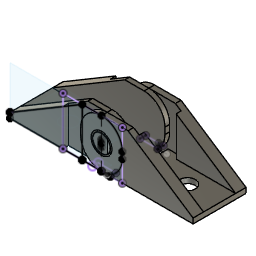
chain-link-ends (Autodesk Fusion 360 design; units mm, degrees)
Autodesk Fusion 360 part; units mm, degrees
note: some values were not read from the file. Set by a fixed rule: which sketch regions a step uses.
sketch "Sketch1" plane through (0, 0, 0) normal (0, 0, 1) x (1, 0, 0)
  line L0 (0, 0) -> (35, 0)
  line L1 (35, 0) -> (35, 16.5)
  line L2 (35, 16.5) -> (0, 16.5)
  line L3 (0, 16.5) -> (0, 0)
  line L4 (0, 14.75) -> (16.5, 14.75)
  line L5 (16.5, 14.75) -> (16.5, 13.25)
  line L6 (16.5, 13.25) -> (35, 13.25)
  line L7 (0, 1.75) -> (16.5, 1.75)
  line L8 (16.5, 1.75) -> (16.5, 3.25)
  line L9 (16.5, 3.25) -> (35, 3.25)
  line L10 (6.5, 16.5) -> (6.5, 0) construction
  line L11 (0, 8.25) -> (35, 8.25) construction
  line L12 (16.5, 14.75) -> (16.5, 16.5) construction
  line L13 (16.5, 1.75) -> (16.5, 0) construction
  line L14 (12.5, 14.75) -> (12.5, 1.75)
  circle A0 centre (25, 8.25) radius 2.5
  dimension "d1" = 35
  dimension "d2" = 16.5
  dimension "d3" = 6.5
  dimension "d4" = 10
  dimension "d5" = 10
  dimension "d7" = 13
  dimension "d9" = 10
  dimension "d10" = 6
  dimension "d11" = 5
  dimension "d12" = 10
  constraint horizontal L0
  constraint vertical L1
  constraint horizontal L2
  constraint vertical L3
  constraint coincident L0.start L3.end
  constraint coincident L3 L4.start
  constraint perpendicular L3 L4
  constraint perpendicular L4 L5
  constraint coincident L1 L6.end
  constraint perpendicular L1 L6
  constraint coincident L3 L7.start
  constraint perpendicular L3 L7
  constraint perpendicular L6 L8
  constraint coincident L1 L9.end
  constraint perpendicular L1 L9
  constraint coincident L2 L10.start
  constraint coincident L0 L10.end
  constraint perpendicular L0 L10
  constraint midpoint L3 L11.start
  constraint midpoint L1 L11.end
  constraint coincident L2 L12.end
  constraint perpendicular L2 L12
  constraint coincident L0 L13.end
  constraint perpendicular L0 L13
  constraint equal L12 L13
  constraint equal L5 L8
  constraint coincident L4 L14.start
  constraint coincident L7 L14.end
  constraint perpendicular L7 L14
  constraint coincident L11 A0.centre
  measures "d1" distance of L0.start L0.end
  measures "d2" distance of L0.start L2.end
  measures "d3" distance of L3 L10
  measures "d4" distance of L5 L10
  measures "d5" distance of L8 L10
  measures "d7" distance of L4 L7
  measures "d9" distance of L6 L9
  measures "d10" distance of L10 L14
  measures "d11" diameter of A0
  measures "d12" distance of L1 A0.centre
extrude "Extrude1" add sketch "Sketch1" along normal blind 1.6 contours L1 L4 L5 L6 L7 L8 L9 L14 makes body 1
extrude "Extrude2" add sketch "Sketch1" along normal blind 15 contours L0 L1 L3 L7 L8 L9 | L1 L2 L3 L4 L5 L6 bodies 1
sketch "Sketch2" plane through (0, 0, 0) normal (0, -1, 0) x (1, 0, 0)
  line L0 (0, 0) -> (35, 0)
  line L1 (35, 0) -> (35, 15)
  line L2 (35, 15) -> (0, 15)
  line L3 (0, 15) -> (0, 0)
  line L4 (0, 8.5) -> (0, 6.5)
  arc A0 (0, 6.5) -> (6.5, 0) centre (6.5, 6.5) ccw
  arc A1 (6.5, 15) -> (0, 8.5) centre (6.5, 8.5) ccw
  line L5 (6.5, 15) -> (14.7505, 15)
  line L6 (14.7505, 15) -> (35, 1.6)
  line L7 (35, 1.6) -> (35, 0)
  line L8 (6.5, 0) -> (35, 0)
  line L9 (0, 0) -> (35, 0)
  circle A2 centre (6.5, 7.5) radius 3.25
  line L10 (22.5, 1.6) -> (27.5, 1.6)
  line L11 (16.5, 1.6) -> (12.5, 1.6)
  line L12 (12.5, 1.6) -> (16.5, 1.6)
  line L13 (16.5, 1.6) -> (35, 1.6)
  line L14 (35, 1.6) -> (16.5, 1.6)
  line L15 (6.5, 0) -> (6.5, 15)
  point P0 (6.5, 0)
  dimension "d17" = 6.5
  constraint coincident L3 L4.start
  constraint coincident L3 L4.end
  constraint coincident L0 P0
  constraint tangent L4 A0
  constraint coincident L2 A1.start
  constraint tangent L4 A1
  constraint coincident L2 L5.end
  constraint parallel L2 L5
  constraint coincident L1 L6.end
  constraint coincident L0.end L1.start
  constraint tangent A0 L9
  constraint tangent A1 L5
  constraint coincident P0 A0.end
  constraint coincident L5 A1.start
  constraint vertical L15
  constraint coincident A2.centre L15
  constraint midpoint A2.centre L15
  constraint equal A0 A1
  constraint coincident L6.end L7.start
  measures "d17" diameter of A2
extrude "Extrude3" cut sketch "Sketch2" against normal up to surface (16.5 mm away) contours L0 L3 A0 L9 | A2 L15 | A2 L15 | L2 L3 A1 | L1 L2 L6 bodies 1
copy_body "Body->Comp1" bodies 1 removing the originals makes body 2 in component "end-1"
sketch "Sketch1 (2)" plane through (0, 0, 0) normal (0, 0, 1) x (1, 0, 0) in component "end-2"
  circle A0 centre (10, 8.25) radius 2.5
  line L0 (0, 8.25) -> (35, 8.25) construction
  line L1 (0, 16.5) -> (0, 0)
  line L2 (16.5, 13.25) -> (35, 13.25)
  line L3 (16.5, 14.75) -> (16.5, 16.5) construction
  line L4 (28.5, 14.75) -> (28.5, 1.75) construction
  line L5 (16.5, 1.75) -> (16.5, 0) construction
  line L6 (16.5, 3.25) -> (35, 3.25)
  line L7 (35, 14.75) -> (16.5, 14.75)
  line L8 (16.5, 14.75) -> (16.5, 15.0527)
  line L9 (16.5, 16.5) -> (16.5, 14.75)
  line L10 (16.5, 16.5) -> (0, 16.5)
  line L11 (16.5, 13.25) -> (0, 13.25)
  line L12 (16.5, 3.25) -> (0, 3.25)
  line L13 (16.5, 1.75) -> (35, 1.75)
  line L14 (16.5, 1.75) -> (16.5, 0)
  line L15 (16.5, 0) -> (0, 0)
  line L16 (35, 14.75) -> (35, 13.25)
  line L17 (35, 14.75) -> (35, 3.25)
  line L18 (35, 14.75) -> (35, 1.75)
  line L19 (22.5, 14.75) -> (22.5, 1.75)
  dimension "d21" = 16.5
  dimension "d26" = 10
  dimension "d28" = 5
  dimension "d31" = 10
  dimension "d32" = 6
  dimension "d33" = 6.5
  constraint vertical L1
  constraint coincident L1.end L15.end
  constraint midpoint L0.start L1
  constraint equal L3 L5
  constraint coincident A0.centre L0
  constraint coincident L3 L8.end
  constraint perpendicular L1 L10
  constraint coincident L1 L11.end
  constraint perpendicular L1 L11
  constraint coincident L1 L12.end
  constraint perpendicular L1 L12
  constraint perpendicular L2 L16
  constraint perpendicular L6 L17
  constraint perpendicular L13 L18
  constraint midpoint L0.end L18
  constraint perpendicular L0 L17
  constraint coincident L4.end L13
  constraint coincident L4.start L7
  constraint perpendicular L4 L7
  constraint coincident L7 L19.start
  constraint coincident L13 L19.end
  constraint perpendicular L13 L19
  measures "d21" distance of L1.start L1.end
  measures "d26" distance of L2 L6
  measures "d28" diameter of A0
  measures "d31" distance of A0.centre L1
  measures "d32" distance of L4 L19
  measures "d33" distance of L4 L18
extrude "Extrude1'" add sketch "Sketch1 (2)" along normal blind 1.6 separate body contours L1 L2 L6 L11 L12 L19 makes body 3 in component "end-2"
extrude "Extrude2'" add sketch "Sketch1 (2)" along normal blind 15 contours L1 L2 L7 L8 L9 L10 L11 L19 | L1 L6 L12 L13 L14 L15 L19 | L2 L7 L16 L17 L18 L19 | L6 L13 L18 L19 bodies 3 in component "end-2"
sketch "Sketch2 (2)" plane through (0, 0, 0) normal (0, -1, 0) x (1, 0, 0) in component "end-2"
  line L0 (0, 0) -> (16.5, 0)
  line L1 (16.5, 0) -> (16.5, 15)
  line L2 (16.5, 15) -> (0, 15)
  line L3 (0, 15) -> (0, 0)
  line L4 (16.5, 0) -> (35, 0)
  line L5 (35, 0) -> (35, 15)
  line L6 (35, 15) -> (16.5, 15)
  line L7 (16.5, 15) -> (16.5, 0)
  line L8 (28.5, 0) -> (28.5, 15) construction
  line L9 (0, 1.6) -> (22.5, 15)
  arc A0 (35, 8.5) -> (28.5, 15) centre (28.5, 8.5) ccw
  line L10 (35, 8.5) -> (35, 6.5)
  arc A1 (28.5, 0) -> (35, 6.5) centre (28.5, 6.5) ccw
  line L11 (22.5, 15) -> (28.5, 15)
  line L12 (28.5, 0) -> (0, 0)
  circle A2 centre (28.5, 7.5) radius 2.75
  line L13 (22.5, 0) -> (22.5, 15)
  point P0 (28.5, 0)
  point P1 (0, 1.6)
  point P2 (22.5, 0)
  dimension "d38" = 5.5
  constraint coincident P0 L8.start
  constraint coincident L6 L8.end
  constraint perpendicular L6 L8
  constraint coincident P1 L9.start
  constraint coincident L6 L9.end
  constraint coincident L5 A0.start
  constraint coincident L5 L10.end
  constraint perpendicular L6 L10
  constraint coincident L4 P0
  constraint tangent L10 A1
  constraint equal A0 A1
  constraint tangent A0 L10
  constraint coincident L0.start L3.end
  constraint tangent A1 L12
  constraint midpoint L8 A2.centre
  constraint coincident P2 L13.start
  constraint coincident L11 L9.end
  constraint vertical L13
  measures "d38" diameter of A2
extrude "Extrude3'" cut sketch "Sketch2 (2)" against normal up to surface (16.5 mm away) contours L1 L2 L3 L7 L9 | L1 L6 L7 L9 | L4 L5 A1 | L5 L6 A0 bodies 3 in component "end-2"
extrude "Extrude4" add sketch "Sketch2 (2)" against normal up to surface (1.75 mm away) contours A2 bodies 3 in component "end-2"
sketch "Sketch3" plane through (0, 14.75, 0) normal (0, 1, 0) x (-1, 0, 0) in component "end-2"
  line L0 (-16.5, 11.4267) -> (-22.5, 15)
  line L1 (-22.5, 15) -> (-28.5, 15)
  arc A0 (-28.5, 15) -> (-35, 8.5) centre (-28.5, 8.5) ccw
  line L2 (-35, 8.5) -> (-35, 6.5)
  arc A1 (-35, 6.5) -> (-28.5, 0) centre (-28.5, 6.5) ccw
  line L3 (-28.5, 0) -> (-16.5, 0)
  line L4 (-16.5, 0) -> (-16.5, 11.4267)
  circle A2 centre (-28.5, 7.5) radius 2.75
extrude "Extrude5" add sketch "Sketch3" along normal up to surface (1.75 mm away) contours A2 bodies 3 in component "end-2"
sketch "Sketch4" plane through (0, 0, 0) normal (0, 0, -1) x (1, 0, 0) in component "end-2"
  line L0 (28.5, -3.25) -> (28.5, -1.75)
  line L1 (28.5, -1.75) -> (16.5, -1.75)
  line L2 (16.5, -1.75) -> (16.5, 0)
  line L3 (16.5, 0) -> (0, 0)
  line L4 (0, 0) -> (0, -16.5)
  line L5 (0, -16.5) -> (16.5, -16.5)
  line L6 (16.5, -16.5) -> (16.5, -14.75)
  line L7 (16.5, -14.75) -> (28.5, -14.75)
  line L8 (28.5, -14.75) -> (28.5, -13.25)
  line L9 (28.5, -13.25) -> (22.5, -13.25)
  line L10 (22.5, -13.25) -> (22.5, -3.25)
  line L11 (22.5, -3.25) -> (28.5, -3.25)
  circle A0 centre (10, -8.25) radius 2.5
  line L12 (31.25, -16.5) -> (25.75, -16.5)
  line L13 (31.25, -14.75) -> (25.75, -14.75)
  line L14 (31.25, 0) -> (25.75, 0)
  line L15 (25.75, -1.75) -> (31.25, -1.75)
  line L16 (31.25, -14.75) -> (29.7816, -16.5)
  line L17 (31.25, -14.75) -> (34.0632, -14.75) construction
  line L18 (25.75, -16.5) -> (25.75, -14.75)
  line L19 (29.7816, -16.5) -> (31.25, -16.5)
  line L20 (31.25, -14.75) -> (31.25, -16.5)
  line L21 (31.25, -1.75) -> (30.2816, 0)
  line L22 (30.2816, 0) -> (31.25, 0)
  line L23 (31.25, 0) -> (31.25, -1.75)
  dimension "d45" = 130
  constraint horizontal L17
  constraint coincident L13.start L16.start
  constraint coincident L12 L16.end
  constraint coincident L12.end L18.start
  constraint coincident L13.end L18.end
  constraint coincident L12.start L19.end
  constraint coincident L15.end L21.start
  constraint coincident L14 L21.end
  constraint coincident L14.start L22.end
  constraint parallel L14 L22
  measures "d45" angle of L16 L17
extrude "Extrude6" cut sketch "Sketch4" against normal up to surface (15 mm away) contours L12 L16 L19 L20 | L14 L21 L22 L23 bodies 3 in component "end-2"
component "end-1" placed x (1, 0, 0) y (0, 1, 0) z (0, 0, 1) at (0, 0, 0)
component "end-2" placed x (1, 0, 0) y (0, 1, 0) z (0, 0, 1) at (-22, 0, 0)
